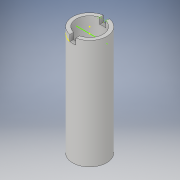
# Autodesk Inventor part: pusher
Saved by Autodesk Inventor 2018 (Build 220112000, 112)
## iProperties
Created: 2019-05-27
Part Number: pusher
Material: Generic
Document SubType Name: Modeling
Designer: Piyush
Density: 1 g/cm^3
Appearance: Default
Author: Piyush
Autodesk Inventor part; units mm, degrees
ref_plane "YZ Plane" through (0, 0, 0) normal (1, 0, 0) x (0, 1, 0)
ref_plane "XZ Plane" through (0, 0, 0) normal (0, 1, 0) x (-1, 0, 0)
ref_plane "XY Plane" through (0, 0, 0) normal (0, 0, 1) x (1, 0, 0)
sketch "Sketch1" plane through (0, 0, 0) normal (0, 1, 0) x (-1, 0, 0)
  point P0 (0, 0)
sketch "Sketch2" plane through (0, 0, 0) normal (0, 1, 0) x (-1, 0, 0)
  circle A0 centre (0, 0) radius 11
  circle A1 centre (0, 0) radius 14
  dimension "d0" = 22
  dimension "d1" = 28
  constraints: 2 centre point, 2 coincident
  measures "d0" diameter of A0
  measures "d1" diameter of A1
extrude "Extrusion1" add sketch "Sketch2" along normal blind 90 contours A0 | A1
hole "Hole1" at (0, 90, 0) direction (0, -1, 0) diameter 22 depth 90 tip angle 118
sketch "Sketch3" plane through (0, 90, 0) normal (0, 1, 0) x (1, 0, 0)
  circle A0 centre (0, 0) radius 11 projected
  circle A1 centre (0, 0) radius 14 projected
  line L0 (2.5, 13.775) -> (2.5, 10.7121)
  line L1 (-2.5, 13.775) -> (-2.5, 10.7121)
  line L2 (-2.5, -10.7121) -> (-2.5, -13.775)
  line L3 (2.5, -10.7121) -> (2.5, -13.775)
  constraints: 8 end point, 8 point on circle, 4 vertical
extrude "Extrusion2" cut sketch "Sketch3" against normal blind 5 contours L3 A1 L2 A0
sketch "Sketch4" plane through (0, 90, 0) normal (0, 1, 0) x (1, 0, 0)
  arc A0 (2.5, -10.7121) -> (-2.5, -10.7121) centre (0, 0) ccw projected
  circle A1 centre (0, 0) radius 14 projected
  line L0 (-2.5, 13.775) -> (-2.5, 10.7121)
  circle A2 centre (0, 0) radius 11 projected
  line L1 (2.5, 13.775) -> (2.5, 10.7121)
  constraints: 4 end point, 4 point on circle, 1 vertical
sketch "Sketch5" plane through (0, 90, 0) normal (0, 1, 0) x (1, 0, 0)
  point P0 (0, 0)
sketch "Sketch6" plane through (0, 90, 0) normal (0, 1, 0) x (1, 0, 0)
  point P0 (0, 0)
extrude "Extrusion3" cut sketch "Sketch4" against normal blind 5 contours A0 L0 A1 L1
sketch "Sketch7" plane through (0, 90, 0) normal (0, 1, 0) x (1, 0, 0)
  point P0 (0, 0)
  point P1 (-2.4887, 10.7148)
  point P2 (2.5, 10.7121)
sketch "Sketch8" plane through (0, 0, 0) normal (0, 1, 0) x (-1, 0, 0)
  arc A0 (2.5, -10.7121) -> (-2.5, -10.7121) centre (0, 0) ccw
  constraints: 2 point on circle, 1 centre point
sketch "Sketch9" plane through (0, 85, 0) normal (0, 1, 0) x (1, 0, 0)
  arc A0 (-2.5, 13.775) -> (-2.5, -13.775) centre (0, 0) ccw projected
  line L0 (-14, 0) -> (14.5387, 0)
  constraints: 2 end point, 1 horizontal, 1 point on circle
body "Solid1"
